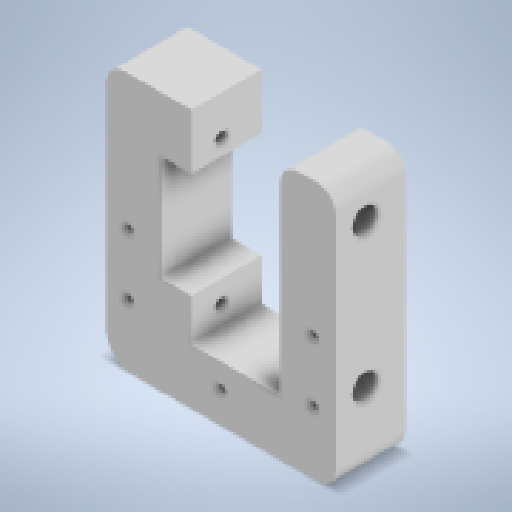
# Autodesk Inventor part: Крепление стрелялки
Saved by Autodesk Inventor 2023.2 (Build 272271030, 271C)
## iProperties
Created: 2024-02-13
Part Number: Крепление стрелялки
Material: Типовые
Document SubType Name: Modeling
Designer: I9232
Density: 1 g/cm^3
Appearance: По умолчанию
Author: I9232
Autodesk Inventor part; units mm, degrees
ref_plane "YZ Plane" through (0, 0, 0) normal (1, 0, 0) x (0, 1, 0)
ref_plane "XZ Plane" through (0, 0, 0) normal (0, 1, 0) x (-1, 0, 0)
ref_plane "XY Plane" through (0, 0, 0) normal (0, 0, 1) x (1, 0, 0)
sketch "Эскиз1" plane through (0, 0, 0) normal (0, 0, 1) x (1, 0, 0)
  line L0 (0, 0) -> (27, 0)
  line L1 (27, 0) -> (27, 22.4859)
  line L2 (12, 15) -> (0, 15)
  line L3 (0, 15) -> (0, 0)
  line L4 (27, 0) -> (21.9283, 0)
  line L5 (12, 15) -> (12, 70)
  line L6 (12, 70) -> (27, 70)
  line L7 (27, 70) -> (27, 0)
  line L8 (0, 0) -> (-35, 0)
  line L9 (-12, 15) -> (0, 15)
  line L10 (-20, 26.4) -> (-20, 55)
  line L11 (-20, 70) -> (-35, 70)
  line L12 (-35, 70) -> (-35, 0)
  line L13 (-12, 15) -> (-12, 26.4)
  line L14 (-12, 26.4) -> (-20, 26.4)
  line L15 (-20, 70) -> (-12, 70)
  line L16 (-12, 70) -> (-12, 55)
  line L17 (-12, 55) -> (-20, 55)
  line L18 (12, 60) -> (12, 70)
  dimension "d37" = 11.4
  dimension "d38" = 8
  dimension "d40" = 15
  dimension "d41" = 70
  dimension "d45" = 12
  constraints: 38 end point, 6 parallel, 5 perpendicular, 3 horizontal
  measures "d37" distance of L9.start L13.end
  measures "d38" distance of L13.end L10.start
  measures "d40" distance of L5.end L6.end
  measures "d41" distance of L11.end L12.end
  measures "d45" distance of L2.start L2.end
extrude "Выдавливание1" add sketch "Эскиз1" along normal blind 14 and the other way blind 5
sketch "Эскиз3" plane through (0, 0, -5) normal (0, 0, -1) x (-1, 0, 0)
  circle A0 centre (28.98, 17) radius 1.25
  circle A1 centre (3.98, 8.5) radius 1.25
  circle A2 centre (-21.02, 17) radius 1.25
  line L0 (-27, 0) -> (35, 0) projected
  circle A3 centre (29, 33.5) radius 1.25
  circle A4 centre (-21, 33.5) radius 1.25
  point P0 (0, 0)
  point P1 (4, 0)
  dimension "d10" = 2.5
  dimension "d12" = 8.5
  dimension "d14" = 50
  dimension "d27" = 17
  dimension "d28" = 25
  dimension "d29" = 17
  dimension "d30" = 25
  constraints: 5 centre point, 4 equal radius, 1 midpoint
  measures "d10" diameter of A0
  measures "d12" distance of point (4, 0) A1.centre
  measures "d14" distance of A4.centre A3.centre
  measures "d27" distance from line of L0 A0.centre
  measures "d28" horizontal distance of A0.centre A1.centre
  measures "d29" distance from line of L0 A2.centre
  measures "d30" horizontal distance of A2.centre A1.centre
extrude "Выдавливание3" cut sketch "Эскиз3" against normal up to surface (19 mm away)
fillet "Сопряжение1" radius 5 4 edges at (27, 0, 4.5) (-35, 70, 4.5) (12, 70, 4.5) (27, 70, 4.5)
sketch "Эскиз5" plane through (-35, 5, -5) normal (-1, 0, 0) x (0, 0, 1)
  circle A0 centre (11, 15.5) radius 1.5 projected
  circle A1 centre (11, 54.5) radius 1.5 projected
  point P0 (5, -5)
extrude "Выдавливание5" cut sketch "Эскиз5" against normal up to surface (23 mm away)
sketch "Эскиз6" plane through (27, 5, 14) normal (1, 0, 0) x (0, 0, -1)
  circle A0 centre (8, 15.5) radius 1.5 projected
  circle A1 centre (8, 54.5) radius 1.5 projected
  point P0 (14, -5)
extrude "Выдавливание6" cut sketch "Эскиз6" against normal up to surface (15 mm away)
sketch "Эскиз7" plane through (27, 5, 14) normal (1, 0, 0) x (0, 0, -1)
  circle A0 centre (8, 15.5) radius 3.5
  circle A1 centre (8, 54.5) radius 3.5
  circle A2 centre (8, 15.5) radius 1.5 construction
  circle A3 centre (8, 54.5) radius 1.5 construction
  point P0 (14, -5)
  dimension "d47" = 7
  constraints: 2 centre point, 2 coincident, 1 equal radius
  measures "d47" diameter of A0
extrude "Выдавливание7" cut sketch "Эскиз7" against normal blind 4
sketch "Эскиз8" plane through (-35, 5, -5) normal (-1, 0, 0) x (0, 0, 1)
  circle A0 centre (11, 15.5) radius 1.5 construction
  circle A1 centre (11, 54.5) radius 1.5 construction
  line L0 (0, 10) -> (19, 10) projected
  circle A2 centre (11, 15.5) radius 3.5
  circle A3 centre (11, 54.5) radius 3.5
  point P0 (5, -5)
  constraints: 2 centre point, 2 coincident
extrude "Выдавливание8" cut sketch "Эскиз8" against normal blind 4
fillet "Сопряжение2" radius 7 1 edges at (-35, 0, 4.5)
